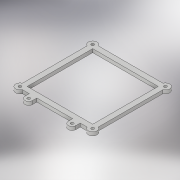
# Autodesk Inventor part: trellisCaptiveBottom
Saved by Autodesk Inventor 2017 (Build 210142000, 142)
## iProperties
Created: 2017-05-22
Part Number: trellisCaptiveBottom
Material: Generic
Document SubType Name: Modeling
Designer: Dominic Gaiero
Density: 1 g/cm^3
Appearance: Default
Author: Dominic Gaiero
Autodesk Inventor part; units mm, degrees
ref_plane "YZ Plane" through (0, 0, 0) normal (1, 0, 0) x (0, 1, 0)
ref_plane "XZ Plane" through (0, 0, 0) normal (0, 1, 0) x (-1, 0, 0)
ref_plane "XY Plane" through (0, 0, 0) normal (0, 0, 1) x (1, 0, 0)
sketch "Sketch1" plane through (0, 0, 0) normal (0, 1, 0) x (-1, 0, 0)
  line L0 (495.455, 411.2754) -> (555.855, 411.2754)
  line L1 (555.855, 411.2754) -> (555.855, 381.0754)
  line L2 (495.455, 381.0754) -> (495.455, 411.2754)
  line L3 (560.655, 416.0754) -> (555.4584, 416.0754)
  line L4 (490.655, 416.0754) -> (490.655, 410.8788)
  line L5 (495.455, 411.2754) -> (490.655, 416.0754)
  line L6 (555.855, 411.2754) -> (560.655, 416.0754)
  line L7 (490.655, 381.0754) -> (560.655, 381.0754)
  arc A0 (556.3458, 411.7662) -> (556.9421, 411.2754) centre (559.1743, 414.5947) ccw
  arc A1 (494.9642, 411.7662) -> (495.8516, 416.0754) centre (492.1358, 414.5947) ccw
  line L8 (560.655, 410.8788) -> (560.655, 416.0754)
  arc A2 (555.4584, 416.0754) -> (555.855, 412.3625) centre (559.1743, 414.5947) ccw
  line L9 (495.8516, 416.0754) -> (490.655, 416.0754)
  line L10 (490.655, 410.8788) -> (490.655, 381.0754)
  arc A3 (490.655, 410.8788) -> (494.9642, 411.7662) centre (492.1358, 414.5947) ccw
  arc A4 (495.8516, 416.0754) -> (490.655, 410.8788) centre (492.1358, 414.5947) ccw
  circle A5 centre (492.1358, 414.5947) radius 1.3
  arc A6 (555.855, 412.3625) -> (556.3458, 411.7662) centre (559.1743, 414.5947) ccw
  arc A7 (560.655, 410.8788) -> (555.4584, 416.0754) centre (559.1743, 414.5947) ccw
  arc A8 (556.9421, 411.2754) -> (560.655, 410.8788) centre (559.1743, 414.5947) ccw
  circle A9 centre (559.1743, 414.5947) radius 1.3
  line L11 (525.655, 416.0754) -> (525.655, 381.0754)
  line L12 (560.655, 381.0754) -> (560.655, 410.8788)
  arc A10 (560.655, 351.272) -> (556.9421, 350.8754) centre (559.1743, 347.5562) ccw
  arc A11 (555.855, 349.7884) -> (555.4584, 346.0754) centre (559.1743, 347.5562) ccw
  line L13 (560.655, 381.0754) -> (560.655, 351.272)
  line L14 (555.855, 350.8754) -> (555.855, 381.0754)
  line L15 (525.655, 346.0754) -> (525.655, 381.0754)
  line L16 (555.4584, 346.0754) -> (495.8516, 346.0754)
  line L17 (495.455, 350.8754) -> (555.855, 350.8754)
  line L18 (495.455, 350.8754) -> (490.655, 346.0754)
  line L19 (490.655, 346.0754) -> (490.655, 351.272)
  line L20 (495.455, 381.0754) -> (495.455, 350.8754)
  line L21 (560.655, 346.0754) -> (555.4584, 346.0754)
  line L22 (555.855, 350.8754) -> (560.655, 346.0754)
  arc A12 (556.3458, 350.3846) -> (555.855, 349.7884) centre (559.1743, 347.5562) ccw
  arc A13 (556.9421, 350.8754) -> (556.3458, 350.3846) centre (559.1743, 347.5562) ccw
  circle A14 centre (559.1743, 347.5562) radius 1.3
  line L23 (560.655, 351.272) -> (560.655, 346.0754)
  arc A15 (555.4584, 346.0754) -> (560.655, 351.272) centre (559.1743, 347.5562) ccw
  circle A16 centre (492.1358, 347.5562) radius 1.3
  line L24 (495.8516, 346.0754) -> (490.655, 346.0754)
  line L25 (490.655, 351.272) -> (490.655, 381.0754)
  arc A17 (494.9642, 350.3846) -> (490.655, 351.272) centre (492.1358, 347.5562) ccw
  arc A18 (490.655, 351.272) -> (495.8516, 346.0754) centre (492.1358, 347.5562) ccw
  arc A19 (495.8516, 346.0754) -> (494.9642, 350.3846) centre (492.1358, 347.5562) ccw
  circle A20 centre (505.655, 420.0664) radius 1.3
  arc A21 (509.155, 420.0664) -> (502.155, 420.0664) centre (505.655, 420.0664) ccw
  line L26 (502.155, 420.0664) -> (502.155, 416.0754)
  line L27 (509.155, 420.0664) -> (509.155, 416.0754)
  circle A22 centre (545.655, 420.0664) radius 1.3
  line L28 (549.155, 420.0664) -> (549.155, 416.0754)
  arc A23 (549.155, 420.0664) -> (542.155, 420.0664) centre (545.655, 420.0664) ccw
  line L29 (542.155, 420.0664) -> (542.155, 416.0754)
  line L30 (502.155, 416.0754) -> (495.8516, 416.0754)
  line L31 (555.4584, 416.0754) -> (549.155, 416.0754)
  line L32 (542.155, 416.0754) -> (509.155, 416.0754)
  point P0 (0, 0)
  point P1 (525.855, 381.2754)
  point P2 (558.255, 413.6754)
  point P3 (493.055, 413.6754)
  point P4 (493.055, 348.4754)
  point P5 (558.255, 348.4754)
  point P6 (525.855, 380.8754)
  dimension "d0" = 4.8
  dimension "d1" = 70
  dimension "d2" = 8
  dimension "d3" = 2.6
  dimension "d4" = 2.6
  dimension "d5" = 33.5192
  dimension "d6" = 33.5192
  dimension "d7" = 2.6
  dimension "d8" = 20
  dimension "d9" = 7
  constraints: 66 end point, 36 point on circle, 26 symmetric about line, 24 centre point, 18 perpendicular, 14 point on line, 6 coincident, 5 parallel, 2 midpoint, 1 horizontal, 12 other
  measures "d0" distance between parallel lines of L0 L3
  measures "d1" distance of L3.start L4.start
  measures "d2" diameter of A1
  measures "d3" diameter of A5
  measures "d4" diameter of A9
  measures "d5" distance from line of L11 A5.centre
  measures "d6" distance from line of L7 A1.centre
  measures "d7" diameter of A20
  measures "d8" distance from line of L11 A20.centre
  measures "d9" diameter of A21
extrude "Extrusion1" add sketch "Sketch1" along normal blind 3.175 contours L5 A1 L30 L26 A21 L27 L32 L11 L0 | L2 L7 L10 A3 L5 | L11 L32 L29 A23 L28 L31 A2 A6 L6 L0 | L20 L18 A17 L25 L7 | A3 L4 L5 A5 | L5 A5 L9 A1 | L6 A0 A8 L12 L7 L1 | L17 L15 L16 A19 L18 | A5 L5 | L5 A5 | L9 L4 A4 | L7 L13 A10 A13 L22 L14 | A6 A2 L3 L6 A9 | L6 A9 L8 A8 A0 | L17 L22 A12 A11 L16 L15 | A17 L18 A16 L19 | L19 L24 A18 | A19 L24 L18 A16 | A9 L6 | L6 A9 | A16 L18 | L18 A16 | L8 L3 A7 | L23 L22 A14 A13 A10 | A15 L21 L23 | L22 A14 L21 A11 A12 | A14 L22 | L22 A14
extrude "Extrusion2" cut sketch "Sketch1" along normal blind 3.175 contours A5 L5 | L5 A5 | A9 L6 | L6 A9 | A16 L18 | L18 A16 | A14 L22 | L22 A14
body "Solid1"
